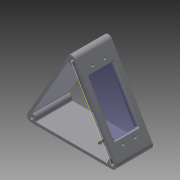
# Autodesk Inventor part: ServoHousing
Saved by Autodesk Inventor 2015 (Build 190159000, 159)
## iProperties
Created: 2014-11-03
Part Number: ServoHousing
Material: Generic
Document SubType Name: Modeling
Designer: rawrdong
Density: 1 g/cm^3
Appearance: Default
Author: rawrdong
Autodesk Inventor part; units mm, degrees
ref_plane "YZ Plane" through (0, 0, 0) normal (1, 0, 0) x (0, 1, 0)
ref_plane "XZ Plane" through (0, 0, 0) normal (0, 1, 0) x (-1, 0, 0)
ref_plane "XY Plane" through (0, 0, 0) normal (0, 0, 1) x (1, 0, 0)
sketch "Sketch2" plane through (0, 0, 0) normal (0, 1, 0) x (-1, 0, 0)
  circle A0 centre (0, 38.1051) radius 1.4
  circle A1 centre (0, 38.1051) radius 3.5
  circle A2 centre (-33, -19.0526) radius 1.4
  circle A3 centre (-33, -19.0526) radius 3.5
  circle A4 centre (33, -19.0526) radius 1.4
  circle A5 centre (33, -19.0526) radius 3.5
  line L0 (-36.0311, -17.3026) -> (-3.0311, 39.8551)
  line L1 (0.5521, 41.5613) -> (-35.7171, -21.2587)
  line L2 (-33, -22.5526) -> (33, -22.5526)
  line L3 (36.0311, -17.3026) -> (3.0311, 39.8551)
  line L4 (-29.7308, -20.3026) -> (29.7308, -20.3026)
  line L5 (32.4479, -15.5964) -> (2.7171, 35.8989)
  line L6 (0, -22.5526) -> (0, -20.3026) construction
  line L7 (19.5311, 11.2763) -> (17.5825, 10.1513) construction
  line L8 (-17.5825, 10.1513) -> (-19.5311, 11.2763) construction
  line L9 (-7.3325, 27.9048) -> (-27.8325, -7.6022) construction
  line L10 (-27.8325, -7.6022) -> (-8.347, -18.8522) construction
  line L11 (-8.347, -18.8522) -> (12.153, 16.6548) construction
  line L12 (12.153, 16.6548) -> (-7.3325, 27.9048) construction
  point P0 (0, 0)
  point P1 (0, 0)
  dimension "d21" = 360
  dimension "d23" = 66
  dimension "d24" = 2.8
  dimension "d25" = 7
  dimension "d30" = 2.25
  dimension "d106" = 22.5
  dimension "d107" = 41
  constraints: 26 end point, 12 point on circle, 7 midpoint, 6 centre point, 6 tangent, 5 parallel, 4 coincident, 2 equal length, 2 point on line, 1 horizontal, 1 perpendicular, 1 vertical alignment, 13 other
  measures "d23" distance of A4.centre A2.centre
  measures "d24" diameter of A2
  measures "d25" diameter of A3
  measures "d30" distance between parallel lines of L0 L1
  measures "d106" distance of L9.end L10.end
  measures "d107" distance of L10.end L11.end
extrude "Extrusion3" add sketch "Sketch2" along normal blind 30 contours A0 L1 A1 | A0 L1 A1 | L1 A3 L0 A1 | L3 A5 L5 A1 | L1 A2 A3 | A3 L1 A2 | A5 | A5 L2 A3 L4
sketch "Servo1" plane through (36.0311, 0, -17.3026) normal (0.8660254, 0, 0.5) x (0.5, 0, -0.8660254)
  line L0 (-66, 30) -> (0, 30) projected
  line L1 (-54, 25.1) -> (-12, 25.1)
  line L2 (-12, 25.1) -> (-12, 4.9)
  line L3 (-12, 4.9) -> (-54, 4.9)
  line L4 (-54, 4.9) -> (-54, 25.1)
  circle A0 centre (-8, 20) radius 1.075
  circle A1 centre (-8, 10) radius 1.075
  line L5 (-33, 30) -> (-33, -15.5284)
  line L6 (-12, 15) -> (-54, 15) construction
  circle A2 centre (-58, 20) radius 1.075
  circle A3 centre (-58, 10) radius 1.075
  line L7 (0, 0) -> (0, 30) projected
  point P0 (-33, 0)
  point P1 (-33, 4.9)
  point P2 (0, 15)
  dimension "d43" = 2.15
  dimension "d44" = 20.2
  dimension "d45" = 42
  dimension "d47" = 50
  dimension "d96" = 10
  constraints: 12 end point, 5 midpoint, 4 centre point, 3 parallel, 3 symmetric about line, 1 equal radius, 1 horizontal, 1 horizontal alignment, 1 perpendicular, 1 point on line, 2 other
  measures "d43" diameter of A0
  measures "d44" distance of L3.end L1.start
  measures "d45" distance of L2.end L3.end
  measures "d47" diameter of A0.centre L5
  measures "d96" distance of A0.centre A1.centre
extrude "Extrusion4" cut sketch "Servo1" against normal blind 25 contours L1 L5 L3 L4 | L1 L2 L3 L5
extrude "Extrusion5" cut sketch "Servo1" against normal up to next contours A0 | A1 | A2 | A3
fillet "Fillet4" radius 0.8 4 edges at (8.0568, 25.1, 28.9003) (8.0568, 4.9, 28.9003) (29.0568, 4.9, -7.4728) (29.0568, 25.1, -7.4728)
ref_plane "Work Plane1" through (2.7171, 0, 35.8989) normal (-0.8660254, 0, -0.5) x (-0.5, 0, 0.8660254)
sketch "Sketch7" plane through (2.7171, 0, 35.8989) normal (-0.8660254, 0, -0.5) x (-0.5, 0, 0.8660254)
  line L0 (-8.7308, 5.7) -> (-8.7308, 24.3) projected
  line L1 (-9.5308, 25.1) -> (-49.9308, 25.1) projected
  arc A0 (-8.7308, 24.3) -> (-9.5308, 25.1) centre (-9.5308, 24.3) ccw projected
  arc A1 (-9.5308, 4.9) -> (-8.7308, 5.7) centre (-9.5308, 5.7) ccw projected
  line L2 (-49.9308, 4.9) -> (-9.5308, 4.9) projected
  arc A2 (-50.7308, 5.7) -> (-49.9308, 4.9) centre (-49.9308, 5.7) ccw projected
  line L3 (-50.7308, 24.3) -> (-50.7308, 5.7) projected
  arc A3 (-49.9308, 25.1) -> (-50.7308, 24.3) centre (-49.9308, 24.3) ccw projected
  line L4 (-49.9308, 27.6) -> (-9.5308, 27.6)
  arc A4 (-6.2308, 24.3) -> (-9.5308, 27.6) centre (-9.5308, 24.3) ccw
  line L5 (-6.2308, 24.3) -> (-6.2308, 5.7)
  arc A5 (-9.5308, 2.4) -> (-6.2308, 5.7) centre (-9.5308, 5.7) ccw
  line L6 (-9.5308, 2.4) -> (-49.9308, 2.4)
  arc A6 (-53.2308, 5.7) -> (-49.9308, 2.4) centre (-49.9308, 5.7) ccw
  line L7 (-53.2308, 5.7) -> (-53.2308, 24.3)
  arc A7 (-49.9308, 27.6) -> (-53.2308, 24.3) centre (-49.9308, 24.3) ccw
  line L8 (-53.2308, 24.3) -> (-62.1767, 24.3)
  line L9 (-62.1767, 24.3) -> (-62.1767, 5.7)
  line L10 (-53.2308, 5.7) -> (-62.1767, 5.7)
  line L11 (-29.7308, 4.9) -> (-29.7308, 25.1) construction
  line L12 (-6.2308, 24.3) -> (2.7151, 24.3)
  line L13 (2.7151, 24.3) -> (2.7151, 5.7)
  line L14 (-6.2308, 5.7) -> (2.7151, 5.7)
  circle A8 centre (-54.7308, 20) radius 1.075 projected
  circle A9 centre (-54.7308, 10) radius 1.075 projected
  circle A10 centre (-4.7308, 10) radius 1.075 projected
  circle A11 centre (-4.7308, 20) radius 1.075 projected
  dimension "d82" = 2.5
  constraints: 22 end point, 8 point on circle, 4 centre point, 3 perpendicular, 2 horizontal, 2 midpoint, 1 vertical, 8 other
  measures "d82" distance between parallel lines of L4 L1
extrude "Extrusion8" add sketch "Sketch7" along normal blind 2
fillet "Fillet6" radius 2 4 edges at (28.4665, 24.3, -10.7003) (4.9665, 24.3, 30.0029) (4.9665, 5.7, 30.0029) (28.4665, 5.7, -10.7003)
chamfer "Chamfer2" distance 2 angle 45 14 edges at (17.5825, 27.6, 10.1513) (6.5619, 27.0386, 29.2396) (5.5864, 24.6403, 30.9292) (3.8728, 24.3, 33.8973) (28.6032, 27.0386, -8.937) (29.5786, 24.6403, -10.6266) (31.2923, 24.3, -13.5947) (17.5825, 2.4, 10.1513) (28.6032, 2.9614, -8.937) (29.5786, 5.3597, -10.6266) (31.2923, 5.7, -13.5947) (6.5619, 2.9614, 29.2396) (5.5864, 5.3597, 30.9292) (3.8728, 5.7, 33.8973)
fillet "Fillet7" radius 0.5 8 edges at (2.7171, 1.8501, 35.8989) (-2.7171, 15, 35.8989) (2.7171, 28.15, 35.8989) (-32.4479, 15, -15.5964) (-29.7308, 15, -20.3026) (29.7308, 15, -20.3026) (32.4479, 1.8501, -15.5964) (32.4479, 28.1499, -15.5964)
chamfer "Chamfer3" distance 0.5 angle 45 8 edges at (19.5311, 4.9, 11.2763) (9.1482, 5.1343, 29.2599) (9.0311, 15, 29.4628) (9.1482, 24.8657, 29.2599) (19.5311, 25.1, 11.2763) (29.9139, 24.8657, -6.7073) (30.0311, 15, -6.9103) (29.9139, 5.1343, -6.7073)
sketch "Sketch9" plane through (33, 0, -22.5526) normal (0, 0, -1) x (-1, 0, 0)
  line L0 (0, 0) -> (0, 30)
  line L1 (17.5, 20) -> (22.5, 20)
  line L2 (22.5, 20) -> (22.5, 10)
  line L3 (22.5, 10) -> (17.5, 10)
  line L4 (17.5, 10) -> (17.5, 20)
  line L5 (0, 15) -> (22.5, 15) construction
  point P0 (-33.5, 0)
  dimension "d97" = 5
  dimension "d98" = 10
  dimension "d104" = 22.5
  constraints: 12 end point, 2 horizontal, 2 midpoint, 2 parallel, 1 perpendicular
  measures "d97" distance of L1.start L1.end
  measures "d98" distance of L3.end L1.start
  measures "d104" distance of L5.start L5.end
extrude "Extrusion9" cut sketch "Sketch9" against normal up to surface surface through (-2.7171, 0, 35.8989) normal (0.8660254, 0, -0.5)
fillet "Fillet8" radius 1.5 4 edges at (10.5, 20, -21.4276) (15.5, 20, -21.4276) (15.5, 10, -21.4276) (10.5, 10, -21.4276)
body "Solid2"
body "Solid3"
